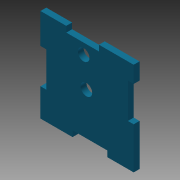
# Autodesk Inventor part: Side A
Saved by Autodesk Inventor 2014 (Build 180170000, 170)
## iProperties
Created: 2014-11-21
Part Number: Side A
Material: Generic
Document SubType Name: Modeling
Designer: JLM
Density: 1 g/cm^3
Appearance: Default
Author: JLM
Autodesk Inventor part; units mm, degrees
ref_plane "YZ Plane" through (0, 0, 0) normal (1, 0, 0) x (0, 1, 0)
ref_plane "XZ Plane" through (0, 0, 0) normal (0, 1, 0) x (-1, 0, 0)
ref_plane "XY Plane" through (0, 0, 0) normal (0, 0, 1) x (1, 0, 0)
sketch "Sketch1" plane through (0, 0, 0) normal (0, 0, 1) x (1, 0, 0)
  line L0 (-25.4, -25.4) -> (25.4, -25.4)
  line L1 (25.4, -25.4) -> (25.4, 25.4)
  line L2 (25.4, 25.4) -> (-25.4, 25.4)
  line L3 (-25.4, 25.4) -> (-25.4, -25.4)
  line L4 (-25.4, -25.4) -> (25.4, 25.4) construction
  line L5 (25.4, -25.4) -> (-25.4, 25.4) construction
  point P0 (0, 0)
  dimension "d0" = 50.8
  dimension "d1" = 50.8
  constraints: 12 end point, 2 midpoint, 2 parallel, 1 horizontal, 1 perpendicular
  measures "d0" distance of L2.end L1.end
  measures "d1" distance of L1.end L0.end
extrude "Extrusion1" add sketch "Sketch1" against normal blind 3.175
sketch "Sketch2" plane through (0, 0, 0) normal (0, 0, 1) x (1, 0, 0)
  line L0 (-13.1551, 25.4) -> (-9.525, 25.4)
  line L1 (-9.525, 25.4) -> (-9.525, 22.225)
  line L2 (-9.525, 22.225) -> (9.525, 22.225)
  line L3 (9.525, 22.225) -> (9.525, 25.4)
  line L4 (-9.525, 25.4) -> (9.525, 25.4)
  line L5 (-9.525, -25.4) -> (9.525, -25.4)
  line L6 (9.525, -25.4) -> (9.525, -22.225)
  line L7 (9.525, -22.225) -> (-9.525, -22.225)
  line L8 (-9.525, -22.225) -> (-9.525, -25.4)
  line L9 (-25.4, 9.525) -> (-22.225, 9.525)
  line L10 (-22.225, 9.525) -> (-22.225, -9.525)
  line L11 (-22.225, -9.525) -> (-25.4, -9.525)
  line L12 (-25.4, -9.525) -> (-25.4, 9.525)
  line L13 (25.4, 9.525) -> (22.225, 9.525)
  line L14 (22.225, 9.525) -> (22.225, -9.525)
  line L15 (22.225, -9.525) -> (25.4, -9.525)
  line L16 (25.4, -9.525) -> (25.4, 9.525)
  line L17 (25.4, -25.4) -> (25.4, 25.4) projected
  line L18 (-25.4, 25.4) -> (-25.4, -25.4) projected
  line L19 (-25.4, -25.4) -> (25.4, -25.4) projected
  line L20 (25.4, 25.4) -> (-25.4, 25.4) projected
  line L21 (-25.4, 25.4) -> (-25.4, -25.4) projected
  dimension "d4" = 3.175
  dimension "d5" = 19.05
  dimension "d17" = 19.05
  dimension "d18" = 3.175
  dimension "d19" = 3.175
  dimension "d20" = 19.05
  dimension "d34" = 3.175
  dimension "d35" = 19.05
  dimension "d47" = 15.875
  dimension "d48" = 15.875
  dimension "d49" = 15.875
  dimension "d50" = 15.875
  dimension "d51" = 15.875
  constraints: 34 end point, 6 parallel, 5 perpendicular, 3 horizontal
  measures "d4" distance of L0.end L1.end
  measures "d5" distance of L1.end L2.end
  measures "d17" distance of L7.end L6.end
  measures "d18" distance of L6.end L5.end
  measures "d19" distance of L10.end L11.end
  measures "d20" distance of L9.end L10.end
  measures "d34" distance of L15.end L14.end
  measures "d35" distance of L14.end L13.end
  measures "d47" distance between parallel lines of L18 L1
  measures "d48" distance between parallel lines of L17 L3
  measures "d49" distance between parallel lines of L20 L9
  measures "d50" distance between parallel lines of L21 L8
  measures "d51" distance between parallel lines of L19 L15
hole "Hole1" at (0, 0, 0) direction (0, 0, -1) diameter 19.05 end through all
extrude "Extrusion3" cut sketch "Sketch2" against normal blind 25.4 contours L4 L3 L2 L1 | L9 L10 L11 L12 | L16 L15 L14 L13 | L8 L7 L6 L5
equation "\"d1\" = d0"
equation "\"d17\" = d5"
equation "\"d18\" = d4"
equation "\"d19\" = d4"
equation "\"d20\" = d5"
equation "\"d34\" = d4"
equation "\"d35\" = d5"
equation "\"d47\" = -0.5 * d5 + 0.5 * d0"
equation "\"d49\" = d47"
equation "\"d50\" = d47"
equation "\"d51\" = d47"
equation "\"d53\" = 0.5 * d0"
body "Solid1"
